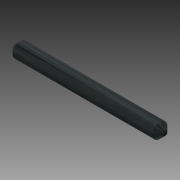
# Autodesk Inventor part: eje17
Saved by Autodesk Inventor 2014 SP1 (Build 180222100, 222)
## iProperties
Created: 2017-09-24
Part Number: eje17
Material: Generic
Document SubType Name: Modeling
Designer: Vivi
Density: 1 g/cm^3
Appearance: Gunmetal - Polished
Author: Vivi
Autodesk Inventor part; units mm, degrees
ref_plane "YZ Plane" through (0, 0, 0) normal (1, 0, 0) x (0, 1, 0)
ref_plane "XZ Plane" through (0, 0, 0) normal (0, 1, 0) x (-1, 0, 0)
ref_plane "XY Plane" through (0, 0, 0) normal (0, 0, 1) x (1, 0, 0)
sketch "Sketch1" plane through (0, 0, 0) normal (1, 0, 0) x (0, 1, 0)
  circle A0 centre (0, 0) radius 1.5
  dimension "d0" = 3
  constraints: 1 centre point, 1 coincident
  measures "d0" diameter of A0
extrude "Extrusion1" add sketch "Sketch1" along normal mid plane 30
chamfer "Chamfer1" distance 1 angle 45 2 edges at (15, -1.5, 0) (-15, -1.5, 0)
body "Solid1"
